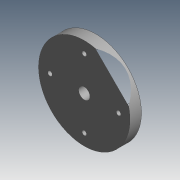
# Autodesk Inventor part: pulleyFlange
Saved by Autodesk Inventor 2015 (Build 190159000, 159)
## iProperties
Created: 2014-09-01
Part Number: pulleyFlange
Material: Generic
Document SubType Name: Modeling
Designer: shohei
Density: 1 g/cm^3
Appearance: Default
Author: shohei
Autodesk Inventor part; units mm, degrees
ref_plane "YZ Plane" through (0, 0, 0) normal (1, 0, 0) x (0, 1, 0)
ref_plane "XZ Plane" through (0, 0, 0) normal (0, 1, 0) x (-1, 0, 0)
ref_plane "XY Plane" through (0, 0, 0) normal (0, 0, 1) x (1, 0, 0)
sketch "Sketch1" plane through (0, 0, 0) normal (0, 1, 0) x (-1, 0, 0)
  circle A0 centre (0, 0) radius 40
  circle A1 centre (30, -0.0076) radius 2
  circle A2 centre (0, 0) radius 5
  arc A3 (-36.0813, 0.572) -> (-36.0815, -0.5576) centre (0, 0) ccw
  arc A4 (-0.0152, -40) -> (-0.0008, -40) centre (0, 0) ccw
  arc A5 (-0.5728, -36.0815) -> (0.5584, -36.0818) centre (0, 0) ccw
  circle A6 centre (0.0076, 30) radius 2
  circle A7 centre (-30, 0.0076) radius 2
  circle A8 centre (-0.0076, -30) radius 2
  point P0 (32, -0.0008)
  point P1 (28.0813, -0.572)
  point P2 (-36.0815, 0.5728)
  point P3 (-0.5576, 36.0815)
  point P4 (0.572, 36.0813)
  point P5 (0.0008, 32)
  point P6 (0.572, 28.0813)
  point P7 (0.5576, -36.0815)
  point P8 (-32, 0.0008)
  point P9 (-28.0813, 0.572)
  point P10 (36.0815, 0.5576)
  point P11 (-0.0008, -32)
  point P12 (-0.572, -28.0813)
  point P13 (-0.5576, 36.0815)
  dimension "d0" = 80
  dimension "d2" = 4
  dimension "d7" = 10
  dimension "d12" = 30
  dimension "d15" = 360
  constraints: 14 point on circle, 9 centre point, 3 coincident, 21 other
  measures "d0" diameter of A0
  measures "d2" diameter of A1
  measures "d7" diameter of A2
  measures "d12" distance of A1.centre A2.centre
extrude "Extrusion2" add sketch "Sketch1" along normal blind 10
body "Solid2"
